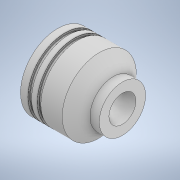
# Autodesk Inventor part: ODSY-0003-103
Saved by Autodesk Inventor 2021 (Build 250183000, 183)
## iProperties
Company: ERPL
Created: 2021-10-21
Part Number: ODSY-0003-103
Material: Generic
Document SubType Name: Modeling
Designer: ALEX CLAY
Density: 2.26577 g/cm^3
Appearance: Default
Project: ODYSSEY
Description: CONICAL NOZZLE INSERT
Authority: CAMERON SEXSMITH
Mass: 1056.87 g
Surface Area: 477.996 cm^2
Volume: 466.45 cm^3
Author: ALEX CLAY
Revision Number: 00
Autodesk Inventor part; units mm, degrees
ref_plane "YZ Plane" through (0, 0, 0) normal (1, 0, 0) x (0, 1, 0)
ref_plane "XZ Plane" through (0, 0, 0) normal (0, 1, 0) x (-1, 0, 0)
ref_plane "XY Plane" through (0, 0, 0) normal (0, 0, 1) x (1, 0, 0)
sketch "Sketch1" plane through (0, 0, 0) normal (0, 0, 1) x (1, 0, 0)
  line L0 (-41.8817, 42.5901) -> (-11.9452, 12.6536)
  line L1 (4.3723, 8.2814) -> (42.5281, 18.5052)
  arc A0 (-11.9452, 12.6536) -> (4.3723, 8.2814) centre (0, 24.5989) ccw
  arc A1 (-41.8817, 42.5901) -> (-46.3719, 44.45) centre (-46.3719, 38.1) ccw
  line L2 (-46.3719, 44.45) -> (-46.3719, 50.8)
  line L3 (-46.3719, 50.8) -> (10.7781, 50.8)
  line L4 (10.7781, 50.8) -> (29.8281, 31.75)
  line L5 (29.8281, 31.75) -> (42.5281, 31.75)
  line L6 (42.5281, 31.75) -> (42.5281, 18.5052)
  line L7 (-25.31, 7.7058) -> (19.1892, 7.7058) construction
  line L8 (-64.1519, 0) -> (60.3081, 0) projected
  point P0 (0, 0)
  dimension "d0" = 57.15
  dimension "d1" = 6.35
  dimension "d2" = 44.45
  dimension "d3" = 50.8
  dimension "d4" = 15
  dimension "d5" = 7.7058
  dimension "d6" = 18.5052
  dimension "d8" = 135
  dimension "d9" = 19.05
  dimension "d13" = 31.75
  dimension "d28" = 45
  constraints: 16 end point, 4 point on circle, 4 tangent, 2 centre point, 2 perpendicular, 2 vertical alignment, 1 horizontal, 1 parallel, 1 vertical
  measures "d0" distance of L2.end L3.end
  measures "d1" radius of A1
  measures "d2" vertical distance of point (0, 0) L2.start
  measures "d3" vertical distance of point (0, 0) L2.end
  measures "d4" angle of L7 L1
  measures "d5" distance from line of point (0, 0) L7
  measures "d6" vertical distance of point (0, 0) L1.end
  measures "d8" angle of L5 L4
  measures "d9" distance between parallel lines of L5 L3
  measures "d13" distance from line of L6 L3.end
  measures "d28" angle of L7 L0
revolve "Revolution1" add sketch "Sketch1" angle 360 about axis through (-10, 0, 0) along (1, 0, 0)
sketch "Sketch3" plane through (0, 0, 0) normal (0, 1, 0) x (-1, 0, 0)
  line L0 (31.297, 50.8) -> (36.0468, 50.8)
  line L1 (36.0468, 50.8) -> (36.0468, 47.9806)
  line L2 (36.0468, 47.9806) -> (31.297, 47.9806)
  line L3 (31.297, 47.9806) -> (31.297, 50.8)
  line L4 (23.3468, 50.8) -> (18.597, 50.8)
  line L5 (18.597, 50.8) -> (18.597, 47.9806)
  line L6 (18.597, 47.9806) -> (23.3468, 47.9806)
  line L7 (23.3468, 47.9806) -> (23.3468, 50.8)
  line L8 (33.6719, 50.8) -> (33.6719, 80.4082) construction
  line L9 (20.9719, 50.8) -> (20.9719, 80.4082) construction
  line L10 (46.3719, 50.8) -> (46.3719, -50.8) projected
  line L11 (54.4041, 0) -> (-9.0674, 0) projected
  point P0 (0, 0)
  dimension "d20" = 12.7
  dimension "d21" = 12.7
  dimension "d22" = 2.8194
  dimension "d23" = 4.7498
  dimension "d24" = 4.7498
  constraints: 20 end point, 4 parallel, 2 collinear, 2 horizontal, 2 midpoint, 2 perpendicular, 2 vertical, 1 point on line
  measures "d20" distance between parallel lines of L8 L10
  measures "d21" distance between parallel lines of L9 L8
  measures "d22" distance of L0.end L1.end
  measures "d23" distance of L0.start L0.end
  measures "d24" distance of L4.start L4.end
revolve "Revolution3" cut sketch "Sketch3" angle 360 about axis through (-10, 0, 0) along (1, 0, 0)
fillet "Fillet1" radius 0.508 4 edges at (-18.597, 0, -47.9806) (-31.297, 0, -47.9806) (-23.3468, 0, -47.9806) (-36.0468, 0, -47.9806)
fillet "Fillet2" radius 0.127 4 edges at (-36.0468, -50.8, 0) (-31.297, -50.8, 0) (-23.3468, -50.8, 0) (-18.597, -50.8, 0)
body "Solid1"
